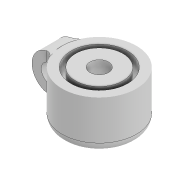
# Autodesk Inventor part: Landing_leg_clamp_large_shoe
Saved by Autodesk Inventor 2022 (Build 260153000, 153)
## iProperties
Created: 2022-07-02
Part Number: Landing_leg_clamp_large_shoe
Material: Generic
Document SubType Name: Modeling
Designer: dell
Density: 1 g/cm^3
Appearance: Default
Author: dell
Autodesk Inventor part; units mm, degrees
ref_plane "YZ Plane" through (0, 0, 0) normal (1, 0, 0) x (0, 1, 0)
ref_plane "XZ Plane" through (0, 0, 0) normal (0, 1, 0) x (-1, 0, 0)
ref_plane "XY Plane" through (0, 0, 0) normal (0, 0, 1) x (1, 0, 0)
sketch "Sketch1" plane through (0, 0, 0) normal (0, 1, 0) x (-1, 0, 0)
  circle A0 centre (0, 0) radius 8
  dimension "d0" = 16
  constraints: 1 centre point, 1 coincident
  measures "d0" diameter of A0
extrude "Extrusion1" add sketch "Sketch1" along normal blind 2.5
sketch "Sketch2" plane through (0, 2.5, 0) normal (0, 1, 0) x (1, 0, 0)
  circle A0 centre (0, 0) radius 5.1
  circle A1 centre (0, 0) radius 6.1
  circle A2 centre (0, 0) radius 8 projected
  circle A3 centre (0, 0) radius 2
  dimension "d3" = 10.2
  dimension "d4" = 12.2
  dimension "d8" = 4
  constraints: 3 centre point, 3 coincident
  measures "d3" diameter of A0
  measures "d4" diameter of A1
  measures "d8" diameter of A3
extrude "Extrusion2" add sketch "Sketch2" along normal blind 8
sketch "Sketch3" plane through (0, 0, 0) normal (0, 0, 1) x (1, 0, 0)
  line L0 (-6.1, 10.5) -> (6.1, 10.5) projected
  line L1 (6.1, 2.5) -> (-6.1, 2.5) projected
  line L2 (6.1, 2.5) -> (-6.1, 2.5) projected
  line L3 (-8, 0) -> (-8, 10.5) projected
  circle A0 centre (-8, 6.5) radius 2
  circle A1 centre (-8, 6.5) radius 4
  line L4 (8, 10.5) -> (-8, 10.5) projected
  line L5 (-6.1, 10.5) -> (-6.1, 2.5) projected
  point P0 (0, 0)
  point P1 (-6.1, 7.1245)
  point P2 (-6.1, 10.0199)
  point P3 (-6.1, 2.9801)
  point P4 (-6.1, 5.8755)
  dimension "d14" = 4
  dimension "d15" = 2
  dimension "d16" = 4
  constraints: 2 centre point, 1 point on line
  measures "d14" diameter of A0
  measures "d15" radial gap between concentric circles of A0 A1
  measures "d16" distance from line of L4 A0.centre
extrude "Extrusion3" add sketch "Sketch3" along normal mid plane 5 contours A1 L3 A0 | L3 A0 L5 A1 | A1 L5 A0 L3
fillet "Fillet2" radius 2 5 edges at (-7.5993, 9.4697, 2.5) (-7.5993, 3.5303, 2.5) (-7.5993, 3.5303, -2.5) (-7.5993, 9.4697, -2.5) (8, 0, 0)
body "Solid1"
